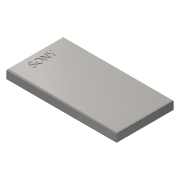
# Autodesk Inventor part: 00_Sony_MDL_Projector
Saved by Autodesk Inventor 2019 (Build 230136000, 136)
## iProperties
Created: 2018-08-23
Part Number: 00_Sony_MDL_Projector
Material: Generisch
Document SubType Name: Modeling
Designer: diederichbenedict
Density: 1 g/cm^3
Appearance: Titan
Author: diederichbenedict
Autodesk Inventor part; units mm, degrees
ref_plane "YZ Plane" through (0, 0, 0) normal (1, 0, 0) x (0, 1, 0)
ref_plane "XZ Plane" through (0, 0, 0) normal (0, 1, 0) x (-1, 0, 0)
ref_plane "XY Plane" through (0, 0, 0) normal (0, 0, 1) x (1, 0, 0)
sketch "Skizze1" plane through (0, 0, 0) normal (0, 0, 1) x (1, 0, 0)
  line L0 (75, 38.65) -> (-75, 38.65)
  line L1 (-75, 38.65) -> (-75, -38.65)
  line L2 (-75, -38.65) -> (75, -38.65)
  line L3 (75, -38.65) -> (75, 38.65)
  line L4 (75, 38.65) -> (-75, -38.65) construction
  line L5 (-75, 38.65) -> (75, -38.65) construction
  point P0 (0, 0)
  dimension "d0" = 150
  dimension "d1" = 77.3
  constraints: 12 end point, 2 midpoint, 2 parallel, 1 horizontal, 1 perpendicular
  measures "d0" distance of L2.end L1.end
  measures "d1" distance of L1.end L0.end
extrude "Extrusion1" add sketch "Skizze1" along normal blind 13.1
fillet "Rundung1" radius 2 8 edges at (0, 38.65, 13.1) (0, 38.65, 0) (0, -38.65, 13.1) (0, -38.65, 0) (75, 0, 13.1) (75, 0, 0) (-75, 0, 13.1) (-75, 0, 0)
sketch "Skizze2" plane through (-75, -38.65, 2) normal (-1, 0, 0) x (0, 0, 1)
  line L0 (0, 0) -> (0, 77.3) projected
  line L1 (0, 0) -> (9.1, 0) projected
  line L2 (9.1, 77.3) -> (9.1, 0) projected
  line L3 (0, 77.3) -> (9.1, 77.3) projected
  circle A0 centre (5.5, 15) radius 5.5
  line L4 (-2, 75.3) -> (-2, 2) projected
  point P0 (-2, 38.65)
  dimension "d5" = 7.5
  dimension "d6" = 15
  constraints: 1 centre point, 1 tangent
  measures "d5" distance from line of A0.centre L4
  measures "d6" distance from line of A0.centre L1
extrude "Extrusion2" cut sketch "Skizze2" against normal blind 13.1 contours A0 L2 | A0 L2
sketch "Skizze3" plane through (-75, 38.65, 2) normal (0, 1, 0) x (1, 0, 0)
  line L0 (13.1, -11) -> (13.1, 0) projected
  line L1 (13.1, -7.4407) -> (35, -7.4407)
  line L2 (35, -7.4407) -> (35, -0.6533)
  line L3 (35, -0.6533) -> (13.1, -0.6533)
  line L4 (13.1, -0.6533) -> (13.1, -7.4407)
  line L5 (50, -7.4407) -> (70, -7.4407)
  line L6 (70, -7.4407) -> (70, -0.6533)
  line L7 (70, -0.6533) -> (50, -0.6533)
  line L8 (50, -0.6533) -> (50, -7.4407)
  line L9 (146.1998, -6.4555) -> (115.5466, -6.4555)
  line L10 (115.5466, -6.4555) -> (115.5466, -0.6533)
  line L11 (115.5466, -0.6533) -> (146.1998, -0.6533)
  line L12 (146.1998, -0.6533) -> (146.1998, -6.4555)
  line L13 (0, 0) -> (0, -9.1) projected
  point P0 (75, 2)
  dimension "d11" = 35
  dimension "d12" = 50
  dimension "d13" = 70
  constraints: 24 end point, 6 parallel, 4 point on line, 3 horizontal, 3 perpendicular
  measures "d11" distance between parallel lines of L2 L13
  measures "d12" distance between parallel lines of L8 L13
  measures "d13" distance between parallel lines of L6 L13
extrude "Extrusion3" cut sketch "Skizze3" against normal blind 13.1
sketch "Skizze4" plane through (0, 0, 13.1) normal (0, 0, 1) x (1, 0, 0)
  line L0 (-67.066, -19.0577) -> (-67.066, 14.3022) construction
  line L1 (-67.066, 14.3022) -> (-57.0354, 14.3022) construction
  line L2 (-57.0354, 14.3022) -> (-57.0354, -19.0577) construction
  line L3 (-57.0354, -19.0577) -> (-67.066, -19.0577) construction
  spline S0 degree 2 poles (-57.0666, -15.3995) (-57.0666, -16.4447) (-57.5034, -17.9111) (-57.8154, -18.5585) knots 0 0 0 1 2 2 2
  line L4 (-57.8154, -18.5585) -> (-59.4221, -18.5585)
  line L5 (-59.4221, -18.5585) -> (-59.4221, -18.4649)
  spline S1 degree 2 poles (-59.4221, -18.4649) (-58.8294, -17.8331) (-58.1742, -16.2341) (-58.1742, -15.4931) knots 0 0 0 1 2 2 2
  spline S2 degree 2 poles (-58.1742, -15.4931) (-58.1742, -14.4324) (-59.0555, -13.3482) (-59.7809, -13.3482) knots 0 0 0 1 2 2 2
  spline S3 degree 2 poles (-59.7809, -13.3482) (-60.3581, -13.3482) (-61.0757, -13.9176) (-61.2551, -14.5338) knots 0 0 0 1 2 2 2
  spline S4 degree 2 poles (-61.2551, -14.5338) (-61.3799, -14.9784) (-61.5515, -15.7193) (-61.6919, -16.2731) knots 0 0 0 1 2 2 2
  spline S5 degree 2 poles (-61.6919, -16.2731) (-61.8245, -16.7723) (-62.2223, -17.5601) (-62.5421, -17.8643) knots 0 0 0 1 2 2 2
  spline S6 degree 2 poles (-62.5421, -17.8643) (-62.8619, -18.1607) (-63.7199, -18.4883) (-64.2814, -18.4883) knots 0 0 0 1 2 2 2
  spline S7 degree 2 poles (-64.2814, -18.4883) (-65.4514, -18.4883) (-67.0348, -16.6631) (-67.0348, -15.2514) knots 0 0 0 1 2 2 2
  spline S8 degree 2 poles (-67.0348, -15.2514) (-67.0348, -14.4402) (-66.715, -13.005) (-66.4108, -12.3888) knots 0 0 0 1 2 2 2
  line L6 (-66.4108, -12.3888) -> (-64.882, -12.3888)
  line L7 (-64.882, -12.3888) -> (-64.882, -12.4824)
  spline S9 degree 2 poles (-64.882, -12.4824) (-65.3032, -12.9426) (-65.9272, -14.3778) (-65.9272, -15.1656) knots 0 0 0 1 2 2 2
  spline S10 degree 2 poles (-65.9272, -15.1656) (-65.9272, -16.0547) (-65.0926, -17.1545) (-64.414, -17.1545) knots 0 0 0 1 2 2 2
  spline S11 degree 2 poles (-64.414, -17.1545) (-63.8057, -17.1545) (-63.0803, -16.5071) (-62.9165, -15.8987) knots 0 0 0 1 2 2 2
  spline S12 degree 2 poles (-62.9165, -15.8987) (-62.8073, -15.4931) (-62.5265, -14.3154) (-62.4095, -13.9254) knots 0 0 0 1 2 2 2
  spline S13 degree 2 poles (-62.4095, -13.9254) (-62.1053, -12.9348) (-60.8807, -12.0144) (-59.9837, -12.0144) knots 0 0 0 1 2 2 2
  spline S14 degree 2 poles (-59.9837, -12.0144) (-59.4143, -12.0144) (-58.3224, -12.4746) (-57.9402, -12.888) knots 0 0 0 1 2 2 2
  spline S15 degree 2 poles (-57.9402, -12.888) (-57.519, -13.3482) (-57.0666, -14.5182) (-57.0666, -15.3995) knots 0 0 0 1 2 2 2
  spline S16 degree 2 poles (-65.7634, -3.9026) (-65.1238, -3.3566) (-63.2519, -2.7482) (-62.0507, -2.7482) knots 0 0 0 1 2 2 2
  spline S17 degree 2 poles (-62.0507, -2.7482) (-60.8807, -2.7482) (-58.9854, -3.341) (-58.3458, -3.9026) knots 0 0 0 1 2 2 2
  spline S18 degree 2 poles (-58.3458, -3.9026) (-57.675, -4.4954) (-57.0354, -6.0631) (-57.0354, -7.0069) knots 0 0 0 1 2 2 2
  spline S19 degree 2 poles (-57.0354, -7.0069) (-57.0354, -7.9819) (-57.6984, -9.5419) (-58.3458, -10.1113) knots 0 0 0 1 2 2 2
  spline S20 degree 2 poles (-58.3458, -10.1113) (-58.9854, -10.665) (-60.8651, -11.2578) (-62.0507, -11.2578) knots 0 0 0 1 2 2 2
  spline S21 degree 2 poles (-62.0507, -11.2578) (-63.2597, -11.2578) (-65.1004, -10.6572) (-65.7634, -10.1035) knots 0 0 0 1 2 2 2
  spline S22 degree 2 poles (-65.7634, -10.1035) (-66.403, -9.5419) (-67.066, -7.9741) (-67.066, -7.0069) knots 0 0 0 1 2 2 2
  spline S23 degree 2 poles (-67.066, -7.0069) (-67.066, -6.0241) (-66.3796, -4.4486) (-65.7634, -3.9026) knots 0 0 0 1 2 2 2
  spline S24 degree 2 poles (-62.0507, -4.082) (-63.0023, -4.082) (-64.4764, -4.4954) (-64.96, -4.8698) knots 0 0 0 1 2 2 2
  spline S25 degree 2 poles (-64.96, -4.8698) (-65.4592, -5.252) (-65.9584, -6.3283) (-65.9584, -6.9991) knots 0 0 0 1 2 2 2
  spline S26 degree 2 poles (-65.9584, -6.9991) (-65.9584, -7.6933) (-65.4748, -8.7385) (-64.96, -9.1363) knots 0 0 0 1 2 2 2
  spline S27 degree 2 poles (-64.96, -9.1363) (-64.4686, -9.5185) (-62.9867, -9.9241) (-62.0507, -9.9241) knots 0 0 0 1 2 2 2
  spline S28 degree 2 poles (-62.0507, -9.9241) (-60.1553, -9.9241) (-58.143, -8.3329) (-58.143, -6.9991) knots 0 0 0 1 2 2 2
  spline S29 degree 2 poles (-58.143, -6.9991) (-58.143, -5.6653) (-60.1553, -4.082) (-62.0507, -4.082) knots 0 0 0 1 2 2 2
  line L8 (-57.2382, 5.543) -> (-57.2382, 4.1078)
  line L9 (-57.2382, 4.1078) -> (-65.5372, -0.1509)
  line L10 (-65.5372, -0.1509) -> (-57.2382, -0.1509)
  line L11 (-57.2382, -0.1509) -> (-57.2382, -1.3442)
  line L12 (-57.2382, -1.3442) -> (-66.8632, -1.3442)
  line L13 (-66.8632, -1.3442) -> (-66.8632, 0.4731)
  line L14 (-66.8632, 0.4731) -> (-59.2427, 4.3496)
  line L15 (-59.2427, 4.3496) -> (-66.8632, 4.3496)
  line L16 (-66.8632, 4.3496) -> (-66.8632, 5.543)
  line L17 (-66.8632, 5.543) -> (-57.2382, 5.543)
  line L18 (-66.8632, 14.232) -> (-61.4969, 10.9795)
  line L19 (-61.4969, 10.9795) -> (-57.2382, 10.9795)
  line L20 (-57.2382, 10.9795) -> (-57.2382, 9.7003)
  line L21 (-57.2382, 9.7003) -> (-61.3643, 9.7003)
  line L22 (-61.3643, 9.7003) -> (-66.8632, 6.4478)
  line L23 (-66.8632, 6.4478) -> (-66.8632, 7.8674)
  line L24 (-66.8632, 7.8674) -> (-62.6279, 10.3477)
  line L25 (-62.6279, 10.3477) -> (-66.8632, 12.8749)
  line L26 (-66.8632, 12.8749) -> (-66.8632, 14.232)
  point P0 (0, 0)
  constraints: 2 other
extrude "Extrusion4" cut sketch "Skizze4" against normal blind 1
